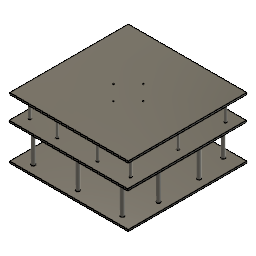
_full structure.1b13a275-2b40-48d6-b8e3-0c061137abb3 (Autodesk Fusion 360 design; units mm, degrees)
Autodesk Fusion 360 part; units mm, degrees
note: some values were not read from the file. Set by a fixed rule: which sketch regions a step uses.
sketch "Sketch2" plane through (0, 0, 0) normal (0, 1, 0) x (1, 0, 0)
  line L0 (100, 100) -> (-100, 100)
  line L1 (-100, 100) -> (-100, -100)
  line L2 (-100, -100) -> (100, -100)
  line L3 (100, -100) -> (100, 100)
  line L4 (100, 100) -> (-100, -100) construction
  line L5 (-100, 100) -> (100, -100) construction
  circle A0 centre (0, -85) radius 3
  circle A1 centre (85, -34) radius 3
  circle A2 centre (75, -85) radius 3
  line L6 (0, -100) -> (0, -75.336)
  line L7 (100, 0) -> (77.1894, 0)
  circle A3 centre (-85, -34) radius 3
  circle A4 centre (0, -85) radius 3
  circle A5 centre (-75, -85) radius 3
  circle A6 centre (85, 34) radius 3
  circle A7 centre (75, 85) radius 3
  circle A8 centre (0, 85) radius 3
  circle A9 centre (-75, 85) radius 3
  circle A10 centre (-85, 34) radius 3
  dimension "d3" = 200
  dimension "d4" = 200
  dimension "d5" = 6
  dimension "d6" = 6
  dimension "d7" = 6
  dimension "d8" = 15
  dimension "d9" = 25
  dimension "d10" = 15
  dimension "d11" = 66
  dimension "d12" = 100
  dimension "d13" = 15
  measures "d3" distance of L0.end L1.end
  measures "d4" distance of L1.end L2.end
  measures "d5" diameter of A0
  measures "d6" diameter of A1
  measures "d7" diameter of A2
  measures "d8" distance of L2 A2.centre
  measures "d9" distance of L3 A2.centre
  measures "d10" distance of L3 A1.centre
  measures "d11" distance of L2 A1.centre
  measures "d12" distance of L1 A0.centre
  measures "d13" distance of L2 A0.centre
extrude "Extrude2" add sketch "Sketch2" along normal blind 3 makes body 1
extrude "Extrude3" add sketch "Sketch2" along normal blind 60 contours A0 L6 A4 | A0 L6 A4 | A1 | A2 | A3 | A5 | A6 | A7 | A8 | A9 | A10 bodies 1
sketch "Sketch3" plane through (0, 0, 0) normal (0, 1, 0) x (1, 0, 0)
  line L0 (100, 100) -> (-100, 100)
  line L1 (-100, 100) -> (-100, -100)
  line L2 (-100, -100) -> (100, -100)
  line L3 (100, -100) -> (100, 100)
  line L4 (100, 100) -> (-100, -100) construction
  line L5 (-100, 100) -> (100, -100) construction
  circle A0 centre (0, -85) radius 2
  circle A1 centre (80, -85) radius 2
  circle A2 centre (85, -34) radius 2
  line L6 (100, 0) -> (78.2297, 0)
  line L7 (0, -100) -> (0, -63.6299)
  circle A3 centre (-80, -85) radius 2
  circle A4 centre (-85, -34) radius 2
  circle A5 centre (-85, 34) radius 2
  circle A6 centre (-80, 85) radius 2
  circle A7 centre (0, 85) radius 2
  circle A8 centre (80, 85) radius 2
  circle A9 centre (85, 34) radius 2
  point P0 (0, -85)
  dimension "d18" = 200
  dimension "d19" = 200
  dimension "d20" = 4
  dimension "d21" = 4
  dimension "d22" = 4
  dimension "d23" = 15
  dimension "d24" = 100
  dimension "d25" = 15
  dimension "d26" = 20
  dimension "d27" = 15
  dimension "d28" = 66
  measures "d18" distance of L0.end L1.end
  measures "d19" distance of L1.end L2.end
  measures "d20" diameter of A0
  measures "d21" diameter of A1
  measures "d22" diameter of A2
  measures "d23" distance of L2 P0
  measures "d24" distance of L3 P0
  measures "d25" distance of L2 A1.centre
  measures "d26" distance of L3 A1.centre
  measures "d27" distance of L3 A2.centre
  measures "d28" distance of L2 A2.centre
extrude "Extrude4" add sketch "Sketch3" along normal blind 3 separate body makes body 2
extrude "Extrude5" add sketch "Sketch3" along normal blind 35 contours A0 L7 | A0 L7 | A1 | A2 | A3 | A4 | A5 | A6 | A7 | A8 | A9 bodies 2
sketch "Sketch4" plane through (0, 0, 0) normal (0, 1, 0) x (1, 0, 0)
  line L0 (100, 100) -> (-100, 100)
  line L1 (-100, 100) -> (-100, -100)
  line L2 (-100, -100) -> (100, -100)
  line L3 (100, -100) -> (100, 100)
  line L4 (100, 100) -> (-100, -100) construction
  line L5 (-100, 100) -> (100, -100) construction
  circle A0 centre (-25, 0) radius 1
  circle A1 centre (0, -25) radius 1
  circle A2 centre (25, 0) radius 1
  circle A3 centre (0, 25) radius 1
  dimension "d33" = 200
  dimension "d34" = 200
  dimension "d37" = 2
  dimension "d38" = 75
  dimension "d39" = 100
  dimension "d41" = 360
  measures "d33" distance of L0.end L1.end
  measures "d34" distance of L1.end L2.end
  measures "d37" diameter of A0
  measures "d38" distance of L1 A0.centre
  measures "d39" distance of L2 A0.centre
extrude "Extrude6" add sketch "Sketch4" along normal blind 3 separate body makes body 3
copy_body "Body->Comp1" bodies 1 removing the originals makes body 4 in component "Component"
copy_body "Body->Comp2" bodies 2 removing the originals makes body 5 in component "Component'"
copy_body "Body->Comp4" bodies 3 removing the originals makes body 6 in component "Component''"
component "Component" placed x (1, 0, 0) y (0, 1, 0) z (0, 0, 1) at (0, 0, 0)
component "Component'" placed x (1, 0, 0) y (0, 1, 0) z (0, 0, 1) at (0, 0, 0)
component "Component''" placed x (1, 0, 0) y (0, 1, 0) z (0, 0, 1) at (0, 0, 0)
